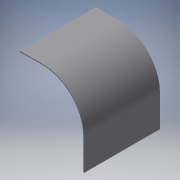
# Autodesk Inventor part: suporte ambu
Saved by Autodesk Inventor 2019 (Build 230136000, 136)
## iProperties
Created: 2020-04-04
Part Number: suporte ambu
Material: Generic
Document SubType Name: Modeling
Designer: Hermann
Density: 1 g/cm^3
Appearance: Default
Author: Hermann
Autodesk Inventor part; units mm, degrees
ref_plane "YZ Plane" through (0, 0, 0) normal (1, 0, 0) x (0, 1, 0)
ref_plane "XZ Plane" through (0, 0, 0) normal (0, 1, 0) x (-1, 0, 0)
ref_plane "XY Plane" through (0, 0, 0) normal (0, 0, 1) x (1, 0, 0)
sketch "Sketch1" plane through (0, 0, 0) normal (0, 0, 1) x (1, 0, 0)
  line L0 (0, 0) -> (0, 50)
  line L1 (-65, 115) -> (-100, 115)
  arc A0 (0, 50) -> (-65, 115) centre (-65, 50) ccw
  dimension "d0" = 65
  dimension "d1" = 50
  dimension "d2" = 100
  constraints: 4 end point, 2 point on circle, 2 tangent, 1 centre point, 1 perpendicular, 1 vertical
  measures "d0" radius of A0
  measures "d1" distance of L0.start L0.end
  measures "d2" distance from line of L0 L1.end
surface extrude "ExtrusionSrf1" sketch "Sketch1" along normal blind 120 shown yes curves L0 A0 L1
thicken "Thicken1" operation new thickness 1.5 both sides no extend neighbours no toward (1, 0, 0) faces at (0, 16.6667, 40) (-39.2548, 109.684, 80) (-76.6667, 115, 40)
body "Solid1"
body "Srf1"
